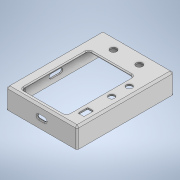
# Autodesk Inventor part: Frontpanel
Saved by Autodesk Inventor 2022 (Build 260153000, 153)
## iProperties
Created: 2020-11-05
Part Number: Frontpanel
Material: Generic
Document SubType Name: Modeling
Designer: simen
Density: 1 g/cm^3
Appearance: Default
Mass: 47.3769 g
Surface Area: 341.342 cm^2
Volume: 47.3769 cm^3
Author: simen
## iProperties of the stored document Frontpanel_3DPrint.ipt
Created: 2022-05-11
Part Number: Frontpanel_3DPrint
Material: Generic
Document SubType Name: Modeling
Designer: simen
Density: 1 g/cm^3
Appearance: Default
Author: simen
Autodesk Inventor part; units mm, degrees
ref_plane "YZ Plane" through (0, 0, 0) normal (1, 0, 0) x (0, 1, 0)
ref_plane "XZ Plane" through (0, 0, 0) normal (0, 1, 0) x (-1, 0, 0)
ref_plane "XY Plane" through (0, 0, 0) normal (0, 0, 1) x (1, 0, 0)
sketch "Sketch1" plane through (0, 0, 0) normal (0, 1, 0) x (-1, 0, 0)
  line L0 (-21.2777, 25.6513) -> (-98.2777, 25.6513)
  line L1 (-98.2777, 25.6513) -> (-98.2777, -79.3487)
  line L2 (-98.2777, -79.3487) -> (-21.2777, -79.3487)
  line L3 (-21.2777, -79.3487) -> (-21.2777, 25.6513)
  point P0 (0, 0)
  dimension "d0" = 77
  dimension "d42" = 105
  constraints: 8 end point, 2 parallel, 1 horizontal, 1 perpendicular
  measures "d0" distance of L2.end L1.end
  measures "d42" distance of L0.end L1.end
extrude "Extrusion1" add sketch "Sketch1" along normal blind 1.5
sketch "Sketch2" plane through (0, 1.5, 0) normal (0, 1, 0) x (1, 0, 0)
  line L0 (26.2777, -20.6513) -> (75.1777, -20.6513)
  line L1 (75.1777, -20.6513) -> (75.1777, 52.7887)
  line L2 (75.1777, 52.7887) -> (26.2777, 52.7887)
  line L3 (26.2777, 52.7887) -> (26.2777, -20.6513)
  line L4 (21.2777, 79.3487) -> (21.2777, -25.6513) projected
  line L5 (21.2777, -25.6513) -> (98.2777, -25.6513) projected
  line L6 (98.2777, 79.3487) -> (21.2777, 79.3487) projected
  point P0 (0, 0)
  dimension "d5" = 5
  dimension "d6" = 5
  dimension "d8" = 48.9
  dimension "d9" = 73.44
  constraints: 8 end point, 2 parallel, 1 horizontal, 1 perpendicular
  measures "d5" distance between parallel lines of L4 L3
  measures "d6" distance between parallel lines of L5 L0
  measures "d8" distance of L0.start L0.end
  measures "d9" distance between parallel lines of L2 L0
extrude "Extrusion2" [suppressed]
sketch "Sketch5" plane through (0, 0, 0) normal (0, -1, 0) x (1, 0, 0)
  line L0 (98.2777, 25.6513) -> (98.2777, -79.3487) projected
  line L1 (21.2777, 25.6513) -> (98.2777, 25.6513) projected
  line L2 (21.2777, -79.3487) -> (21.2777, 25.6513) projected
  line L3 (98.2777, -79.3487) -> (21.2777, -79.3487) projected
  line L4 (96.7777, 24.1513) -> (96.7777, -77.8487)
  line L5 (96.7777, -77.8487) -> (22.7777, -77.8487)
  line L6 (22.7777, -77.8487) -> (22.7777, 24.1513)
  line L7 (22.7777, 24.1513) -> (96.7777, 24.1513)
  point P0 (0, 0)
  dimension "d26" = 1.5
  constraints: 8 end point, 3 other
  measures "d26" distance between parallel lines of L1 L7
extrude "Extrusion7" add sketch "Sketch5" along normal blind 20.5
chamfer "Chamfer2" [suppressed]
fillet "Fillet2" radius 2 4 edges at (21.2777, -9.5, -79.3487) (98.2777, -9.5, -79.3487) (98.2777, -9.5, 25.6513) (21.2777, -9.5, 25.6513)
sketch "Sketch8" plane through (21.2777, -20.5, -77.3487) normal (-1, 0, 0) x (0, 0, 1)
  line L0 (55.5, 8) -> (45.5, 8) construction
  line L1 (55.5, 10.5) -> (45.5, 10.5)
  line L2 (45.5, 5.5) -> (55.5, 5.5)
  arc A0 (55.5, 5.5) -> (55.5, 10.5) centre (55.5, 8) ccw
  arc A1 (45.5, 10.5) -> (45.5, 5.5) centre (45.5, 8) ccw
  line L3 (101, 0) -> (0, 0) projected
  line L4 (101, 0) -> (0, 0) construction
  line L5 (46.4736, 0) -> (44.5264, 16) construction
  line L6 (0, 22) -> (101, 22) projected
  line L7 (0, 22) -> (101, 22) construction
  line L8 (0, 0) -> (0, 22) construction
  circle A2 centre (50.054, 8.1268) radius 1.7526 projected
  line L9 (101, 22) -> (101, 0) projected
  line L10 (0, 0) -> (0, 22) projected
  point P0 (50.5, 8)
  point P1 (50.5, 8)
  dimension "d51" = 10
  dimension "d52" = 5
  dimension "d282" = 14
  constraints: 10 end point, 4 point on circle, 4 tangent, 2 centre point, 2 midpoint, 1 coincident, 1 horizontal, 1 parallel, 1 point on line
  measures "d51" distance of L0.end L0.start
  measures "d52" diameter of A1
  measures "d282" distance from line of L6 point (50.5, 8)
extrude "Extrusion9" cut sketch "Sketch8" against normal blind 10 contours A0 L2 A1 L1 | A2
sketch "Sketch9" plane through (0, 1.5, 0) normal (0, 1, 0) x (1, 0, 0)
  line L0 (35.2777, -20.1513) -> (78.2777, -20.1513)
  line L1 (81.2777, -17.1513) -> (81.2777, 49.8487)
  line L2 (78.2777, 52.8487) -> (35.2777, 52.8487)
  line L3 (32.2777, 49.8487) -> (32.2777, -17.1513)
  arc A0 (32.2777, -17.1513) -> (35.2777, -20.1513) centre (35.2777, -17.1513) ccw
  arc A1 (78.2777, -20.1513) -> (81.2777, -17.1513) centre (78.2777, -17.1513) ccw
  arc A2 (81.2777, 49.8487) -> (78.2777, 52.8487) centre (78.2777, 49.8487) ccw
  arc A3 (35.2777, 52.8487) -> (32.2777, 49.8487) centre (35.2777, 49.8487) ccw
  line L4 (98.2777, -25.6513) -> (98.2777, 79.3487) projected
  line L5 (21.2777, -25.6513) -> (98.2777, -25.6513) projected
  line L6 (22.7777, -24.1513) -> (22.7777, 77.8487) projected
  point P0 (0, 0)
  point P1 (81.2777, 52.8487)
  point P2 (81.2777, -20.1513)
  point P3 (32.2777, 52.8487)
  point P4 (98.2777, -23.6513)
  point P5 (98.2777, 77.3487)
  point P6 (23.2777, -25.6513)
  point P7 (96.2777, -25.6513)
  dimension "d56" = 49
  dimension "d57" = 73
  dimension "d60" = 3
  dimension "d116" = 17
  dimension "d144" = 5.5
  dimension "d283" = 9.5
  constraints: 8 end point, 8 point on circle, 8 tangent, 6 point on line, 4 centre point, 3 equal radius, 2 parallel, 1 horizontal, 1 perpendicular
  measures "d56" distance of point (32.278, 52.849) point (81.278, 52.849)
  measures "d57" distance of point (81.278, 52.849) point (81.278, -20.151)
  measures "d60" radius of A0
  measures "d116" distance between parallel lines of L4 L1
  measures "d144" distance between parallel lines of L5 L0
  measures "d283" distance between parallel lines of L6 L3
extrude "Extrusion10" cut sketch "Sketch9" against normal blind 10
chamfer "Chamfer4" distance 1 angle 45 8 edges at (33.1563, 1.5, 19.2726) (32.2777, 1.5, -16.3487) (33.1563, 1.5, -51.9701) (56.7777, 1.5, -52.8487) (80.399, 1.5, -51.9701) (81.2777, 1.5, -16.3487) (80.399, 1.5, 19.2726) (56.7777, 1.5, 20.1513)
chamfer "Chamfer5" distance 2 angle 45 8 edges at (98.2777, 1.5, -26.8487) (97.6919, 1.5, -78.763) (59.7777, 1.5, -79.3487) (21.8635, 1.5, -78.763) (21.2777, 1.5, -26.8487) (21.8635, 1.5, 25.0655) (59.7777, 1.5, 25.6513) (97.6919, 1.5, 25.0655)
fillet "Fillet3" [suppressed]
sketch "Sketch10" plane through (0, 1.5, 0) normal (0, 1, 0) x (1, 0, 0)
  arc A0 (31.2777, -17.1513) -> (35.2777, -21.1513) centre (35.2777, -17.1513) ccw projected
  line L0 (31.2777, 49.8487) -> (31.2777, -17.1513) projected
  arc A1 (35.2777, 53.8487) -> (31.2777, 49.8487) centre (35.2777, 49.8487) ccw projected
  line L1 (78.2777, 53.8487) -> (35.2777, 53.8487) projected
  arc A2 (82.2777, 49.8487) -> (78.2777, 53.8487) centre (78.2777, 49.8487) ccw projected
  line L2 (82.2777, -17.1513) -> (82.2777, 49.8487) projected
  arc A3 (78.2777, -21.1513) -> (82.2777, -17.1513) centre (78.2777, -17.1513) ccw projected
  line L3 (35.2777, -21.1513) -> (78.2777, -21.1513) projected
  line L4 (96.2777, -23.6513) -> (23.2777, -23.6513) projected
  line L5 (96.2777, 77.3487) -> (96.2777, -23.6513) projected
  line L6 (23.2777, 77.3487) -> (96.2777, 77.3487) projected
  line L7 (23.2777, -23.6513) -> (23.2777, 77.3487) projected
  arc A4 (78.2777, -21.1513) -> (82.2777, -17.1513) centre (78.2777, -17.1513) ccw projected
  line L8 (82.2777, -17.1513) -> (96.2777, -17.1513) construction
  line L9 (89.2777, -17.1513) -> (89.2777, -7.1513) construction
  circle A5 centre (89.2777, -7.1513) radius 2
  line L10 (89.2777, -7.1513) -> (89.2777, 17.8487) construction
  circle A6 centre (89.2777, 17.8487) radius 2
  point P0 (0, 0)
  dimension "d70" = 10
  dimension "d71" = 4
  dimension "d72" = 25
  dimension "d73" = 4
  constraints: 6 end point, 2 centre point, 2 coincident, 2 perpendicular, 1 collinear, 1 midpoint, 1 point on line
  measures "d70" distance of L9.start L9.end
  measures "d71" diameter of A5
  measures "d72" distance of L10.start L10.end
  measures "d73" diameter of A6
extrude "Extrusion11" [suppressed]
sketch "Sketch11" plane through (0, 0, 0) normal (0, -1, 0) x (1, 0, 0)
  arc A0 (90.8777, 20.7513) -> (93.3777, 18.2513) centre (93.3777, 20.7513) ccw
  line L0 (96.7777, 24.1513) -> (96.7777, -77.8487) projected
  line L1 (22.7777, 24.1513) -> (96.7777, 24.1513) projected
  arc A1 (93.3777, -71.9487) -> (90.8777, -74.4487) centre (93.3777, -74.4487) ccw
  arc A2 (28.6777, -74.4487) -> (26.1777, -71.9487) centre (26.1777, -74.4487) ccw
  arc A3 (26.1777, 18.2513) -> (28.6777, 20.7513) centre (26.1777, 20.7513) ccw
  line L2 (96.7777, -77.8487) -> (22.7777, -77.8487) projected
  line L3 (22.7777, -77.8487) -> (22.7777, 24.1513) projected
  line L4 (26.1777, 18.2513) -> (22.7777, 18.2513)
  line L5 (28.6777, 20.7513) -> (28.6777, 24.1513)
  line L6 (26.1777, -71.9487) -> (22.7777, -71.9487)
  line L7 (22.7777, 24.1513) -> (22.7777, -77.8487) projected
  line L8 (28.6777, -74.4487) -> (28.6777, -77.8487)
  line L9 (22.7777, -77.8487) -> (96.7777, -77.8487) projected
  line L10 (90.8777, -74.4487) -> (90.8777, -77.8487)
  line L11 (93.3777, -71.9487) -> (96.7777, -71.9487)
  line L12 (96.7777, -77.8487) -> (96.7777, 24.1513) projected
  line L13 (93.3777, 18.2513) -> (96.7777, 18.2513)
  line L14 (90.8777, 20.7513) -> (90.8777, 25.3811)
  line L15 (96.7777, 24.1513) -> (22.7777, 24.1513) projected
  point P0 (0, 0)
  point P1 (96.7777, 22.1513)
  point P2 (96.7777, -75.8487)
  point P3 (24.7777, 24.1513)
  point P4 (94.7777, 24.1513)
  point P5 (94.7777, -77.8487)
  point P6 (24.7777, -77.8487)
  point P7 (22.7777, -75.8487)
  point P8 (22.7777, 22.1513)
  point P9 (90.8777, -77.8487)
  point P10 (90.8777, 24.1513)
  dimension "d117" = 5
  dimension "d118" = 3.4
  dimension "d119" = 3.4
  dimension "d120" = 5
  dimension "d121" = 5
  dimension "d122" = 5
  dimension "d123" = 3.4
  dimension "d124" = 3.4
  dimension "d125" = 3.4
  dimension "d126" = 3.4
  dimension "d127" = 3.4
  dimension "d128" = 3.4
  constraints: 16 end point, 8 perpendicular, 8 point on circle, 8 tangent, 7 point on line, 4 centre point
  measures "d117" diameter of A0
  measures "d118" distance from line of L0 A0.centre
  measures "d119" distance from line of L1 A0.centre
  measures "d120" diameter of A1
  measures "d121" diameter of A2
  measures "d122" diameter of A3
  measures "d123" distance from line of L0 A1.centre
  measures "d124" distance from line of L2 A1.centre
  measures "d125" distance from line of L2 A2.centre
  measures "d126" distance from line of L3 A2.centre
  measures "d127" distance from line of L1 A3.centre
  measures "d128" distance from line of L3 A3.centre
extrude "Extrusion13" add sketch "Sketch11" along normal blind 17 contours L14 L1 L0 L13 A0 | L5 A3 L4 L3 L1 | L0 L2 L10 A1 L11 | L6 A2 L8 L2 L3
sketch "Sketch14" plane through (93.3777, -17, 20.7513) normal (0, -1, 0) x (-0.7071068, 0, 0.7071068)
  arc A0 (1.7678, 1.7678) -> (-1.7678, 1.7678) centre (0, 0) ccw projected
  arc A1 (-65.5488, 65.5488) -> (-65.5488, 69.0843) centre (-67.3166, 67.3166) ccw projected
  arc A2 (-21.5668, 113.0664) -> (-18.0312, 113.0664) centre (-19.799, 114.8341) ccw projected
  arc A3 (45.7498, 49.2853) -> (45.7498, 45.7498) centre (47.5176, 47.5176) ccw projected
  line L0 (45.7498, 45.7498) -> (48.154, 43.3456) projected
  line L1 (52.3259, 47.5176) -> (48.154, 43.3456) projected
  line L2 (48.154, 51.6895) -> (52.3259, 47.5176) projected
  line L3 (48.154, 51.6895) -> (45.7498, 49.2853) projected
  circle A4 centre (48.9318, 47.5176) radius 2
  line L4 (-18.0312, 113.0664) -> (-15.6271, 115.4705) projected
  line L5 (-19.799, 119.6425) -> (-15.6271, 115.4705) projected
  line L6 (-23.9709, 115.4705) -> (-19.799, 119.6425) projected
  line L7 (-23.9709, 115.4705) -> (-21.5668, 113.0664) projected
  line L8 (-65.5488, 69.0843) -> (-67.953, 71.4885) projected
  line L9 (-72.1249, 67.3166) -> (-67.953, 71.4885) projected
  line L10 (-67.953, 63.1446) -> (-72.1249, 67.3166) projected
  line L11 (-67.953, 63.1446) -> (-65.5488, 65.5488) projected
  line L12 (-1.7678, 1.7678) -> (-4.1719, -0.6364) projected
  line L13 (0, -4.8083) -> (-4.1719, -0.6364) projected
  line L14 (4.1719, -0.6364) -> (0, -4.8083) projected
  line L15 (4.1719, -0.6364) -> (1.7678, 1.7678) projected
  circle A5 centre (-19.799, 116.2484) radius 2
  circle A6 centre (-68.7308, 67.3166) radius 2
  circle A7 centre (0, -1.4142) radius 2
  point P0 (51.3546, 80.7013)
  dimension "d303" = 4
  dimension "d306" = 3.5
  dimension "d307" = 3.5
  dimension "d308" = 4
  dimension "d309" = 3.5
  dimension "d310" = 3.5
  dimension "d311" = 3.5
  dimension "d312" = 3.5
  dimension "d313" = 4
  dimension "d315" = 3.5
  dimension "d316" = 3.5
  dimension "d317" = 4
  constraints: 4 centre point
  measures "d303" diameter of A4
  measures "d306" distance from line of L0 A4.centre
  measures "d307" distance from line of L3 A4.centre
  measures "d308" diameter of A5
  measures "d309" distance from line of L7 A5.centre
  measures "d310" distance from line of L4 A5.centre
  measures "d311" distance from line of A6.centre L8
  measures "d312" distance from line of L11 A6.centre
  measures "d313" diameter of A7
  measures "d315" distance from line of L12 A7.centre
  measures "d316" distance from line of L15 A7.centre
  measures "d317" diameter of A6
extrude "Extrusion15" cut sketch "Sketch14" against normal blind 4 contours A4 | A5 | A6 | A7
sketch "Sketch15" plane through (0, 0, 0) normal (0, -1, 0) x (1, 0, 0)
  circle A0 centre (92.7777, 15.1513) radius 3.5
  circle A1 centre (26.7777, 15.1513) radius 3.5
  line L0 (22.7777, 24.1513) -> (96.7777, 24.1513) projected
  line L1 (96.7777, 24.1513) -> (96.7777, -77.8487) projected
  line L2 (22.7777, -77.8487) -> (22.7777, 24.1513) projected
  circle A2 centre (26.7777, -65.8487) radius 3.5
  circle A3 centre (92.7777, -65.8487) radius 3.5
  point P0 (0, 0)
  point P1 (24.7777, 24.1513)
  point P2 (94.7777, 24.1513)
  point P3 (96.7777, 22.1513)
  point P4 (96.7777, -75.8487)
  point P5 (22.7777, -75.8487)
  point P6 (22.7777, 22.1513)
  dimension "d145" = 7
  dimension "d146" = 7
  dimension "d147" = 9
  dimension "d148" = 9
  dimension "d149" = 4
  dimension "d150" = 4
  dimension "d151" = 7
  dimension "d152" = 7
  dimension "d153" = 4
  dimension "d154" = 4
  dimension "d155" = 90
  dimension "d156" = 90
  dimension "d166" = 66
  constraints: 4 centre point
  measures "d145" diameter of A0
  measures "d146" diameter of A1
  measures "d147" distance from line of L0 A0.centre
  measures "d148" distance from line of L0 A1.centre
  measures "d149" distance from line of L1 A0.centre
  measures "d150" distance from line of L2 A1.centre
  measures "d151" diameter of A2
  measures "d152" diameter of A3
  measures "d153" distance from line of L1 A3.centre
  measures "d154" distance from line of L2 A2.centre
  measures "d155" distance from line of L0 A2.centre
  measures "d156" distance from line of L0 A3.centre
  measures "d166" distance of A1.centre A0.centre
extrude "Extrusion16" add sketch "Sketch15" along normal blind 6.65
sketch "Sketch17" plane through (23.2777, -20.5, 25.6513) normal (0, 0, 1) x (1, 0, 0)
  line L0 (0, 20) -> (73, 20) projected
  line L1 (73, 0) -> (0, 0) projected
  line L2 (33.5, 10.5) -> (39.5, 10.5) construction
  line L3 (33.5, 8.5) -> (39.5, 8.5)
  line L4 (39.5, 12.5) -> (33.5, 12.5)
  arc A0 (33.5, 12.5) -> (33.5, 8.5) centre (33.5, 10.5) ccw
  arc A1 (39.5, 8.5) -> (39.5, 12.5) centre (39.5, 10.5) ccw
  line L5 (33.305, 9.08) -> (39.695, 9.08) projected
  arc A2 (39.695, 9.08) -> (40.97, 10.355) centre (39.695, 10.355) ccw projected
  arc A3 (33.305, 12.04) -> (32.23, 10.965) centre (33.305, 10.965) ccw projected
  arc A4 (32.03, 10.355) -> (33.305, 9.08) centre (33.305, 10.355) ccw projected
  arc A5 (39.695, 9.08) -> (40.97, 10.355) centre (39.695, 10.355) ccw projected
  arc A6 (40.67, 10.965) -> (39.695, 11.94) centre (39.695, 10.965) ccw projected
  line L6 (0, 0) -> (0, 20) projected
  line L7 (73, 20) -> (73, 0) projected
  point P0 (-23.2777, 20.5)
  point P1 (36.5, 10.5)
  dimension "d167" = 6
  dimension "d168" = 4
  dimension "d169" = 9.5
  dimension "d170" = 10.5
  constraints: 8 end point, 4 point on circle, 4 tangent, 2 centre point, 1 horizontal, 1 midpoint, 1 parallel
  measures "d167" distance of L2.start L2.end
  measures "d168" diameter of A1
  measures "d169" distance between parallel lines of L0 L2
  measures "d170" distance from line of L1 point (36.5, 10.5)
extrude "Extrusion17" cut sketch "Sketch17" against normal blind 4 contours A0 L4 A1 L3
chamfer "Chamfer6" distance 1 angle 45 4 edges at (59.7777, -8, 25.6513) (64.7777, -10, 25.6513) (59.7777, -12, 25.6513) (54.7777, -10, 25.6513)
sketch "Sketch18" plane through (0, 1.5, 0) normal (0, 1, 0) x (1, 0, 0)
  line L0 (96.2777, 77.3487) -> (96.2777, -23.6513) projected
  line L1 (82.2777, -17.1513) -> (96.2777, -17.1513)
  line L2 (81.2777, 49.8487) -> (82.2777, 49.8487) projected
  line L3 (96.7777, -24.1513) -> (96.7777, 77.8487) projected
  circle A0 centre (88.7777, 21.3487) radius 3.25
  circle A1 centre (88.7777, 40.3987) radius 3.25
  line L4 (96.2777, -23.6513) -> (23.2777, -23.6513) projected
  point P0 (0, 0)
  point P1 (96.7777, -22.1513)
  point P2 (96.7777, 75.8487)
  point P3 (97.2777, 77.3487)
  point P4 (97.2777, -26.6513)
  dimension "d178" = 6.5
  dimension "d179" = 6.5
  dimension "d191" = 7.5
  dimension "d192" = 7.5
  dimension "d275" = 19.05
  dimension "d276" = 45
  constraints: 2 centre point, 2 end point, 1 horizontal, 2 other
  measures "d178" diameter of A0
  measures "d179" diameter of A1
  measures "d275" distance of A1.centre A0.centre
  measures "d276" distance from line of L4 A0.centre
extrude "Extrusion18" cut sketch "Sketch18" against normal blind 10
sketch "Sketch19" plane through (0, 1.5, 0) normal (0, 1, 0) x (1, 0, 0)
  circle A0 centre (88.7777, 40.3987) radius 3.25 projected
  circle A1 centre (88.7777, 21.3487) radius 3.25 projected
  arc A2 (31.2777, -17.1513) -> (35.2777, -21.1513) centre (35.2777, -17.1513) ccw projected
  line L0 (31.2777, 49.8487) -> (31.2777, -17.1513) projected
  arc A3 (35.2777, 53.8487) -> (31.2777, 49.8487) centre (35.2777, 49.8487) ccw projected
  line L1 (78.2777, 53.8487) -> (35.2777, 53.8487) projected
  arc A4 (82.2777, 49.8487) -> (78.2777, 53.8487) centre (78.2777, 49.8487) ccw projected
  line L2 (82.2777, -17.1513) -> (82.2777, 49.8487) projected
  arc A5 (78.2777, -21.1513) -> (82.2777, -17.1513) centre (78.2777, -17.1513) ccw projected
  line L3 (35.2777, -21.1513) -> (78.2777, -21.1513) projected
  line L4 (96.2777, -23.6513) -> (23.2777, -23.6513) projected
  line L5 (96.2777, 77.3487) -> (96.2777, -23.6513) projected
  line L6 (23.2777, 77.3487) -> (96.2777, 77.3487) projected
  line L7 (23.2777, -23.6513) -> (23.2777, 77.3487) projected
  arc A6 (35.2777, 53.8487) -> (31.2777, 49.8487) centre (35.2777, 49.8487) ccw projected
  arc A7 (82.2777, 49.8487) -> (78.2777, 53.8487) centre (78.2777, 49.8487) ccw projected
  line L8 (23.2777, 77.3487) -> (96.2777, 77.3487) projected
  circle A8 centre (73.7777, 66.3487) radius 3.5
  line L9 (96.2777, 77.3487) -> (96.2777, -23.6513) projected
  line L10 (81.2777, -17.1513) -> (81.2777, 49.8487) projected
  line L11 (88.7777, 40.3987) -> (88.7777, 73.4928)
  line L12 (96.7777, 75.8487) -> (96.7777, -22.1513) projected
  line L13 (24.7777, 77.8487) -> (94.7777, 77.8487) projected
  line L14 (82.2777, -17.1513) -> (82.2777, 49.8487) projected
  line L15 (82.2777, 43.5388) -> (96.2777, 43.5388)
  line L16 (87.0277, -12.4013) -> (91.5277, -12.4013)
  line L17 (92.5277, -11.4013) -> (92.5277, -2.9013)
  line L18 (91.5277, -1.9013) -> (87.0277, -1.9013)
  line L19 (86.0277, -2.9013) -> (86.0277, -11.4013)
  line L20 (86.0277, -12.4013) -> (92.5277, -1.9013) construction
  line L21 (92.5277, -12.4013) -> (86.0277, -1.9013) construction
  arc A9 (86.0277, -11.4013) -> (87.0277, -12.4013) centre (87.0277, -11.4013) ccw
  arc A10 (91.5277, -12.4013) -> (92.5277, -11.4013) centre (91.5277, -11.4013) ccw
  arc A11 (92.5277, -2.9013) -> (91.5277, -1.9013) centre (91.5277, -2.9013) ccw
  arc A12 (87.0277, -1.9013) -> (86.0277, -2.9013) centre (87.0277, -2.9013) ccw
  line L22 (77.1824, 60.8487) -> (70.6824, 71.3487) construction
  line L23 (35.0277, 59.5987) -> (41.5277, 70.0987) construction
  line L24 (98.2777, -23.6513) -> (98.2777, 77.3487) projected
  circle A13 centre (45.7777, 66.3487) radius 3.5
  line L25 (22.7777, -24.1513) -> (96.7777, -24.1513) projected
  point P0 (0, 0)
  point P1 (86.949, 59.6109)
  point P2 (88.2777, 58.5987)
  point P3 (89.2777, -7.1513)
  point P4 (98.2777, -25.6513)
  point P5 (98.2777, 79.3487)
  dimension "d184" = 7
  dimension "d200" = 10.5
  dimension "d201" = 1
  dimension "d207" = 6.5
  dimension "d209" = 5.75
  dimension "d277" = 7
  dimension "d278" = 28
  dimension "d284" = 11
  dimension "d285" = 11
  dimension "d286" = 22.5
  dimension "d318" = 17
  constraints: 20 end point, 11 point on line, 8 point on circle, 8 tangent, 6 centre point, 3 equal radius, 3 perpendicular, 2 parallel, 1 horizontal, 1 midpoint
  measures "d184" diameter of A8
  measures "d200" distance of L20.end L21.start
  measures "d201" radius of A9
  measures "d207" distance between parallel lines of L17 L19
  measures "d209" distance between parallel lines of L24 L17
  measures "d277" diameter of A13
  measures "d278" distance of A13.centre A8.centre
  measures "d284" distance from line of L6 A8.centre
  measures "d285" distance from line of L6 A13.centre
  measures "d286" distance from line of A13.centre L7
  measures "d318" distance from line of point (89.278, -7.151) L25
extrude "Extrusion19" cut sketch "Sketch19" against normal up to surface (1.5 mm away) contours A8 | A9 L19 A12 L18 A11 L17 A10 L16 | A13
sketch "Sketch23" plane through (94.7777, -20.5, 24.1513) normal (0, 0, -1) x (-1, 0, 0)
  line L0 (72, 0) -> (-2, 0) projected
  arc A0 (38, 8.5) -> (38, 12.5) centre (38, 10.5) ccw projected
  line L1 (40, 10.5) -> (40, 2)
  arc A1 (32, 12.5) -> (32, 8.5) centre (32, 10.5) ccw projected
  line L2 (30, 10.5) -> (30, 2)
  line L3 (30, 2) -> (40, 2)
  line L4 (3.9, 20.5) -> (66.1, 20.5) projected
  line L5 (-2, 3.5) -> (-2, 0) projected
  line L6 (72, 3.5) -> (72, 0) projected
  line L7 (66.1, 3.5) -> (66.1, 20.5) projected
  line L8 (72, 3.5) -> (66.1, 3.5) projected
  line L9 (3.9, 20.5) -> (3.9, 3.5) projected
  line L10 (3.9, 3.5) -> (-2, 3.5) projected
  point P0 (94.7777, 20.5)
  dimension "d241" = 2
  constraints: 6 end point, 2 point on circle, 2 tangent, 2 vertical
  measures "d241" distance between parallel lines of L0 L3
extrude "Extrusion23" [suppressed]
chamfer "Chamfer9" [suppressed]
sketch "Sketch28" plane through (92.7777, -6.65, 15.1513) normal (0, -1, 0) x (-0.9891866, 0, 0.1466627)
  arc A0 (1.1526, -3.3048) -> (-1.1526, -3.3048) centre (0, 0) ccw projected
  circle A1 centre (-11.8797, 80.1241) radius 3.5 projected
  circle A2 centre (53.4066, 89.8039) radius 3.5 projected
  arc A3 (67.3482, 6.8516) -> (65.1422, 6.1827) centre (65.2863, 9.6797) ccw projected
  circle A4 centre (65.2863, 9.6797) radius 2
  circle A5 centre (0, 0) radius 2
  circle A6 centre (-11.8797, 80.1241) radius 2
  circle A7 centre (53.4066, 89.8039) radius 2
  point P0 (89.5523, 28.5944)
  dimension "d294" = 4
  dimension "d295" = 4
  dimension "d296" = 4
  dimension "d297" = 4
  constraints: 4 centre point, 4 coincident
  measures "d294" diameter of A4
  measures "d295" diameter of A5
  measures "d296" diameter of A6
  measures "d297" diameter of A7
extrude "Extrusion26" cut sketch "Sketch28" against normal blind 5 contours A4 | A5 | A6 | A7
chamfer "Chamfer12" distance 0.5 angle 45 8 edges at (28.756, -6.65, 14.8579) (94.756, -6.65, -66.1421) (28.756, -6.65, -66.1421) (94.756, -6.65, 14.8579) (26.5919, -17, 20.337) (95.7919, -17, 20.337) (95.7919, -17, -76.863) (26.5919, -17, -76.863)
sketch "Sketch29" plane through (0, 0, 0) normal (0, -1, 0) x (1, 0, 0)
  line L0 (28.7777, -2.8487) -> (25.7777, -2.8487)
  line L1 (25.7777, -2.8487) -> (25.7777, -52.8487)
  line L2 (25.7777, -52.8487) -> (28.7777, -52.8487)
  line L3 (28.7777, -52.8487) -> (28.7777, -2.8487)
  line L4 (22.7777, 18.2513) -> (22.7777, -71.9487) projected
  line L5 (22.7777, 18.2513) -> (22.7777, 21.0513) projected
  line L6 (22.7777, 21.0513) -> (22.7777, 22.4513) projected
  line L7 (22.7777, 22.4513) -> (22.7777, 24.1513) projected
  line L8 (22.7777, -77.8487) -> (22.7777, 24.1513) projected
  line L9 (22.7777, -77.8487) -> (22.7777, -76.1487) projected
  line L10 (22.7777, -76.1487) -> (22.7777, -74.7487) projected
  line L11 (22.7777, -74.7487) -> (22.7777, -71.9487) projected
  line L12 (22.7777, -31.8487) -> (22.7777, -21.8487) projected
  line L13 (22.7777, -21.8487) -> (22.7777, -21.8487) projected
  line L14 (22.7777, -21.8487) -> (22.7777, -31.8487) projected
  line L15 (22.7777, -31.8487) -> (22.7777, -31.8487) projected
  line L16 (28.6777, -77.8487) -> (90.8777, -77.8487) projected
  line L17 (87.2777, -47.8487) -> (84.2777, -47.8487)
  line L18 (84.2777, -47.8487) -> (84.2777, -52.8487)
  line L19 (84.2777, -52.8487) -> (87.2777, -52.8487)
  line L20 (87.2777, -52.8487) -> (87.2777, -47.8487)
  line L21 (96.7777, 24.1513) -> (96.7777, -77.8487) projected
  line L22 (87.2777, 20.6513) -> (84.2777, 20.6513)
  line L23 (84.2777, 20.6513) -> (84.2777, 15.6513)
  line L24 (84.2777, 15.6513) -> (87.2777, 15.6513)
  line L25 (87.2777, 15.6513) -> (87.2777, 20.6513)
  line L26 (96.2777, 23.6513) -> (23.2777, 23.6513) projected
  point P0 (0, 0)
  dimension "d320" = 6
  dimension "d321" = 3
  dimension "d322" = 50
  dimension "d323" = 25
  dimension "d326" = 25
  dimension "d327" = 5
  dimension "d328" = 12.5
  dimension "d329" = 3
  dimension "d339" = 5
  dimension "d340" = 3
  constraints: 24 end point, 7 equal length, 3 horizontal, 3 perpendicular, 2 collinear
  measures "d320" distance between parallel lines of L4 L3
  measures "d321" distance between parallel lines of L3 L1
  measures "d322" distance between parallel lines of L2 L0
  measures "d323" distance between parallel lines of L16 L2
  measures "d326" distance between parallel lines of L16 L19
  measures "d327" distance between parallel lines of L19 L17
  measures "d328" distance between parallel lines of L21 L18
  measures "d329" distance between parallel lines of L18 L20
  measures "d339" distance between parallel lines of L24 L22
  measures "d340" distance between parallel lines of L26 L22
extrude "Extrusion27" add sketch "Sketch29" along normal blind 3
chamfer "Chamfer13" distance 1.5 angle 45 3 edges at (84.2777, -3, -50.3487) (28.7777, -3, -27.8487) (84.2777, -3, 18.1513)
sketch "Sketch31" plane through (96.7777, -20.5, 24.1513) normal (0, 0, -1) x (-1, 0, 0)
  line L0 (68.1, 3.5) -> (68.1, 20.5) projected
  line L1 (69.3446, 13.85) -> (69.3446, 20.5) projected
  line L2 (71.6248, 13.85) -> (69.3446, 13.85) projected
  line L3 (71.6248, 20.5) -> (71.6248, 13.85) projected
  line L4 (69.3446, 20.5) -> (71.6248, 20.5) projected
  line L5 (66.5, 20.5) -> (66.5, 13.85) projected
  line L6 (70.6, 13.85) -> (69.3446, 13.85) projected
  line L7 (71.6248, 13.85) -> (70.6, 13.85) projected
  line L8 (71.6248, 13.85) -> (69.3446, 13.85) projected
  line L9 (67.5, 13.85) -> (72.5, 13.85) projected
  line L10 (66.5, 13.85) -> (73.5, 13.85) projected
  line L11 (66.5, 17.1127) -> (68.1, 17.1127)
  line L12 (5.9, 20.5) -> (68.1, 20.5) projected
  line L13 (66.5, 20.5) -> (68.1, 20.5)
  line L14 (68.1, 20.5) -> (66.5, 20.5)
  point P0 (96.7777, 20.5)
  constraints: 6 end point, 2 perpendicular, 2 point on line, 1 horizontal, 1 other
extrude "Extrusion28" cut sketch "Sketch31" along normal blind 14.1125 contours L11 L5 L12 L0
chamfer "Chamfer14" distance 1.5 angle 45 1 edges at (30.2777, -3.3873, 15.1513)
sketch "Sketch33" plane through (96.7777, -20.5, -77.8487) normal (-1, 0, 0) x (0, 0, 1)
  line L0 (89.5, 20.5) -> (89.5, 13.85) projected
  line L1 (96.4381, 20.5) -> (96.4381, 13.85) projected
  line L2 (90.25, 20.5) -> (96.4381, 20.5) projected
  line L3 (89.5116, 20.5) -> (90.25, 20.5) projected
  line L4 (96.1, 20.5) -> (89.5116, 20.5) projected
  line L5 (96.1, 13.85) -> (96.1, 20.5) projected
  line L6 (96.4381, 13.85) -> (96.1, 13.85) projected
  line L7 (91, 19.7) -> (91, 20.5) projected
  line L8 (5.9, 20.5) -> (96.1, 20.5) projected
  line L9 (92.039, 20.5) -> (89.5, 17.0455)
  point P0 (77.8487, 20.5)
  constraints: 2 end point, 2 point on line
extrude "Extrusion29" cut sketch "Sketch33" along normal blind 9.35 contours L8 L3 L2 L9 L0
body "Solid1"
